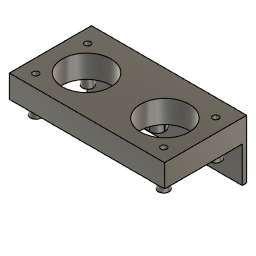
Chassis F360 (Autodesk Fusion 360 archive; units mm, degrees)
design "HC-SR04-UltrasonicSensor v7_Fitted Holes v8"
Autodesk Fusion 360 part; units mm, degrees
ref_plane "WorkPlane1" through (-22.725, -10, 13.61) normal (0, 0, 1) x (1, 0, 0)
sketch "Sketch1" plane through (0, 0, 13.61) normal (0, 0, 1) x (1, 0, 0)
  circle A0 centre (13.12, 0) radius 8
  circle A1 centre (-13.12, 0) radius 8
  circle A2 centre (-13.12, 0) radius 8.12
  circle A3 centre (13.12, 0) radius 8.12
  line L0 (26, -13) -> (-26, -13)
  line L1 (-26, -13) -> (-26, 13)
  line L2 (-26, 13) -> (26, 13)
  line L3 (26, 13) -> (26, -13)
  line L4 (26, -13) -> (-26, 13) construction
  line L5 (-26, -13) -> (26, 13) construction
  constraint concentric A1 A2
  constraint concentric A0 A3
  constraint horizontal L0
  constraint perpendicular L0 L1
  constraint parallel L0 L2
  constraint parallel L1 L3
  constraint coincident L4 origin
  constraint coincident L5 origin
extrude "Extrude1" add sketch "Sketch1" against normal blind 7.62 contours L0 L1 L2 L3
sketch "Sketch2" plane through (0, 0, 5.99) normal (0, 0, -1) x (-1, 0, 0)
  circle A0 centre (13.12, 0) radius 8.12
  circle A1 centre (-13.12, 0) radius 8.12
  line L0 (26, 13) -> (-26, 13)
  line L1 (-26, 13) -> (-26, -13)
  line L2 (-26, -13) -> (26, -13)
  line L3 (26, -13) -> (26, 13)
  arc A2 (5, 7.4356) -> (3.2, 9.2356) centre (3.2, 7.4356) ccw
  line L4 (5, 7.4356) -> (5, 7.3356)
  arc A3 (3.2, 5.5356) -> (5, 7.3356) centre (3.2, 7.3356) ccw
  line L5 (-3.2, 9.2356) -> (3.2, 9.2356)
  line L6 (3.2, 5.5356) -> (-3.2, 5.5356)
  arc A4 (-5, 7.3356) -> (-3.2, 5.5356) centre (-3.2, 7.3356) ccw
  line L7 (-5, 7.3356) -> (-5, 7.4356)
  arc A5 (-3.2, 9.2356) -> (-5, 7.4356) centre (-3.2, 7.4356) ccw
  line L8 (3.2, 9.2356) -> (-3.2, 9.2356)
  line L9 (3.2, 5.5356) -> (-3.2, 5.5356)
  arc A6 (5, 7.4356) -> (3.2, 9.2356) centre (3.2, 7.4356) ccw
  arc A7 (-3.2, 9.2356) -> (-5, 7.4356) centre (-3.2, 7.4356) ccw
  line L10 (5, 7.4356) -> (5, 7.3356)
  arc A8 (3.2, 5.5356) -> (5, 7.3356) centre (3.2, 7.3356) ccw
  arc A9 (-5, 7.3356) -> (-3.2, 5.5356) centre (-3.2, 7.3356) ccw
  line L11 (-5, 7.4356) -> (-5, 7.3356)
  line L12 (-5.1, 7.4356) -> (-5.1, 7.3356)
  arc A10 (-5.1, 7.3356) -> (-3.2, 5.4356) centre (-3.2, 7.3356) ccw
  line L13 (3.2, 5.4356) -> (-3.2, 5.4356)
  arc A11 (3.2, 5.4356) -> (5.1, 7.3356) centre (3.2, 7.3356) ccw
  line L14 (5.1, 7.4356) -> (5.1, 7.3356)
  arc A12 (5.1, 7.4356) -> (3.2, 9.3356) centre (3.2, 7.4356) ccw
  line L15 (3.2, 9.3356) -> (-3.2, 9.3356)
  arc A13 (-3.2, 9.3356) -> (-5.1, 7.4356) centre (-3.2, 7.4356) ccw
  line L16 (-5.7, 7.4356) -> (-5.7, 7.3356)
  arc A14 (-5.7, 7.3356) -> (-3.2, 4.8356) centre (-3.2, 7.3356) ccw
  line L17 (3.2, 4.8356) -> (-3.2, 4.8356)
  arc A15 (3.2, 4.8356) -> (5.7, 7.3356) centre (3.2, 7.3356) ccw
  line L18 (5.7, 7.4356) -> (5.7, 7.3356)
  arc A16 (5.7, 7.4356) -> (3.2, 9.9356) centre (3.2, 7.4356) ccw
  line L19 (3.2, 9.9356) -> (-3.2, 9.9356)
  arc A17 (-3.2, 9.9356) -> (-5.7, 7.4356) centre (-3.2, 7.4356) ccw
  circle A18 centre (21.425, -8.7) radius 1
  circle A19 centre (-21.425, -8.7) radius 1
  circle A20 centre (-21.425, 8.7) radius 1
  circle A21 centre (21.425, 8.7) radius 1
  circle A22 centre (-21.425, -8.7) radius 1.8
  circle A23 centre (-21.425, 8.7) radius 1.8
  circle A24 centre (21.425, 8.7) radius 1.8
  circle A25 centre (21.425, -8.7) radius 1.8
  point P0 (0, 7.3856)
  point P1 (0, 7.3856)
  dimension "d130" = 0.1
  dimension "d131" = 0.7
  dimension "d8" = 3.6
  dimension "d9" = 3.6
  dimension "d10" = 3.6
  dimension "d11" = 3.6
  dimension "d14" = 2
  dimension "d15" = 2
  dimension "d16" = 2
  dimension "d17" = 2
  constraint concentric A2 A6
  constraint concentric A5 A7
  constraint coincident A2.end L5.end
  constraint coincident L5.start A5.start
  constraint coincident A3.start L6.start
  constraint coincident L6.end A4.end
  constraint coincident A2.start L4.start
  constraint coincident L4.end A3.end
  constraint tangent L6 A8
  constraint tangent L4 A8
  constraint tangent L6 A9
  constraint tangent L7 A9
  constraint coincident L7.end A5.end
  constraint tangent A4 L11
  constraint coincident P1 P0
  constraint concentric A20 A23
  constraint concentric A21 A24
  constraint concentric A18 A25
  measures "d130" distance of L11
  measures "d8" diameter of A22
  measures "d9" diameter of A23
  measures "d10" diameter of A24
  measures "d11" diameter of A25
  measures "d14" diameter of A20
  measures "d15" diameter of A21
  measures "d16" diameter of A18
  measures "d17" diameter of A19
extrude "Extrude2" add sketch "Sketch2" along normal blind 3.69 contours L16 A14 L17 A15 L18 A16 L19 A17
sketch "Sketch3" plane through (0, 0, 5.99) normal (0, 0, -1) x (-1, 0, 0)
extrude "Extrude4" cut sketch "Sketch2" against normal through all contours A18 | A19 | A20 | A21
extrude "Extrude6" add sketch "Sketch2" along normal blind 4.38 contours A22 | A23 | A24 | A25
sketch "Sketch4" plane through (0, 13, 0) normal (0, 1, 0) x (-1, 0, 0)
  line L0 (26, 13.61) -> (-26, 13.61)
  line L1 (-26, 13.61) -> (-26, 5.99)
  line L2 (-26, 5.99) -> (26, 5.99)
  line L3 (26, 5.99) -> (26, 13.61)
  line L4 (26, -6.01) -> (-26, -6.01)
  line L5 (-26, -6.01) -> (-26, 25.61)
  line L6 (-26, 25.61) -> (26, 25.61)
  line L7 (26, 25.61) -> (26, -6.01)
  line L8 (5, 5.99) -> (21.24, 5.99)
  dimension "d18" = 12
  dimension "d19" = 12
  constraint horizontal L4
  constraint vertical L5
  constraint horizontal L6
  constraint vertical L7
  measures "d18" distance of L4 L8
  measures "d19" distance of L0 L6
extrude "Extrude7" add sketch "Sketch4" along normal blind 1.5
extrude "Extrude8" cut 1 faces at (8.6667, 13.5, 25.61) along direction (0, 0, -1) up to surface (12 mm away)

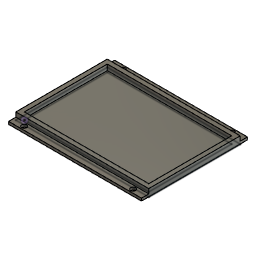
design "BreadBoard Mount"
Autodesk Fusion 360 part; units mm, degrees
sketch "Sketch1" plane through (0, 0, 0) normal (0, 1, 0) x (1, 0, 0)
  line L0 (0, 0) -> (87, 0)
  line L1 (87, 0) -> (87, 58)
  line L2 (87, 58) -> (0, 58)
  line L3 (0, 58) -> (0, 0)
  line L4 (-3, 61) -> (90, 61)
  line L5 (90, 61) -> (90, -3)
  line L6 (90, -3) -> (-3, -3)
  line L7 (-3, -3) -> (-3, 61)
  dimension "d1" = 87
  dimension "d2" = 58
  dimension "d3" = 3
  dimension "d4" = 3
  dimension "d5" = 3
  dimension "d6" = 3
  constraint horizontal L0
  constraint vertical L1
  constraint horizontal L2
  constraint vertical L3
  constraint coincident L0.start L3.end
  constraint horizontal L4
  constraint vertical L5
  constraint horizontal L6
  constraint vertical L7
  measures "d1" distance of L0.start L0.end
  measures "d2" distance of L0.start L2.end
  measures "d3" distance of L1 L5
  measures "d4" distance of L0 L6
  measures "d5" distance of L3 L7
  measures "d6" distance of L2 L4
extrude "Extrude1" add sketch "Sketch1" along normal blind 5
extrude "Extrude2" add sketch "Sketch1" along normal blind 1 contours L0 L1 L2 L3
sketch "Sketch2" plane through (0, 0, 0) normal (0, 1, 0) x (1, 0, 0)
  line L0 (90, -3) -> (-3, -3)
  line L1 (-3, -3) -> (-3, 61)
  line L2 (-3, 61) -> (90, 61)
  line L3 (90, 61) -> (90, -3)
  circle A0 centre (81.6, 63.54) radius 1.75
  circle A1 centre (5.4, 63.54) radius 1.75
  line L4 (-3, -3) -> (-3, 61)
  line L5 (-3, 61) -> (90, 61)
  circle A2 centre (81.6, -5.54) radius 1.75
  circle A3 centre (5.4, -5.54) radius 1.75
  line L6 (90, -3) -> (-3, -3)
  line L7 (-3, 66.08) -> (90, 66.08)
  line L8 (90, 66.08) -> (90, -8.08)
  line L9 (90, -8.08) -> (-3, -8.08)
  line L10 (-3, -8.08) -> (-3, 66.08)
  dimension "d11" = 3.5
  dimension "d12" = 3.5
  dimension "d13" = 76.2
  dimension "d14" = 8.4
  dimension "d15" = 2.54
  dimension "d16" = 3.5
  dimension "d17" = 3.5
  dimension "d18" = 2.54
  dimension "d19" = 2.54
  dimension "d21" = 2.54
  dimension "d22" = 2.54
  constraint horizontal L7
  constraint vertical L8
  constraint horizontal L9
  constraint vertical L10
  measures "d11" diameter of A0
  measures "d12" diameter of A1
  measures "d13" distance of A0.centre A1.centre
  measures "d14" distance of A1.centre L4
  measures "d15" distance of A0.centre L5
  measures "d16" diameter of A2
  measures "d17" diameter of A3
  measures "d18" distance of A3.centre L6
  measures "d19" distance of A2.centre L6
  measures "d21" distance of A3.centre L9
  measures "d22" distance of A0.centre L7
extrude "Extrude3" add sketch "Sketch2" along normal blind 1.778 contours L0 L6 L8 L9 L10 | L2 L5 L7 L8 L10
equation "d4 = d3"
equation "d5 = d4"

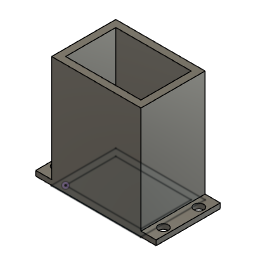
design "NewBatteryMount"
Autodesk Fusion 360 part; units mm, degrees
sketch "Sketch1" plane through (0, 0, 0) normal (0, 1, 0) x (1, 0, 0)
  line L0 (0, 0) -> (27, 0)
  line L1 (27, 0) -> (27, 18)
  line L2 (27, 18) -> (0, 18)
  line L3 (0, 18) -> (0, 0)
  line L4 (-2.5, 20.5) -> (29.5, 20.5)
  line L5 (29.5, 20.5) -> (29.5, -2.5)
  line L6 (29.5, -2.5) -> (-2.5, -2.5)
  line L7 (-2.5, -2.5) -> (-2.5, 20.5)
  dimension "d1" = 27
  dimension "d2" = 18
  dimension "d3" = 2.5
  dimension "d4" = 2.5
  dimension "d5" = 2.5
  dimension "d6" = 2.5
  constraint horizontal L0
  constraint vertical L1
  constraint horizontal L2
  constraint vertical L3
  constraint coincident L0.start L3.end
  constraint horizontal L4
  constraint vertical L5
  constraint horizontal L6
  constraint vertical L7
  measures "d1" distance of L0.start L0.end
  measures "d2" distance of L0.start L2.end
  measures "d3" distance of L0 L6
  measures "d4" distance of L1 L5
  measures "d5" distance of L3 L7
  measures "d6" distance of L2 L4
extrude "Extrude1" add sketch "Sketch1" along normal blind 40
extrude "Extrude2" add sketch "Sketch1" along normal blind 2.5 contours L0 L1 L2 L3
sketch "Sketch2" plane through (0, 0, 0) normal (0, 1, 0) x (1, 0, 0)
  circle A0 centre (-5.6754, 2.65) radius 1.75
  circle A1 centre (32.4246, 2.65) radius 1.75
  line L0 (29.5, -2.5) -> (-2.5, -2.5)
  circle A2 centre (-5.6754, 15.35) radius 1.75
  circle A3 centre (32.4246, 15.35) radius 1.75
  line L1 (29.5, -2.5) -> (-2.5, -2.5)
  line L2 (-2.5, -2.5) -> (-2.5, 20.5)
  line L3 (-2.5, 20.5) -> (29.5, 20.5)
  line L4 (29.5, 20.5) -> (29.5, -2.5)
  line L5 (-8.2154, -2.5) -> (34.9646, -2.5)
  line L6 (34.9646, -2.5) -> (34.9646, 20.5)
  line L7 (34.9646, 20.5) -> (-8.2154, 20.5)
  line L8 (-8.2154, 20.5) -> (-8.2154, -2.5)
  dimension "d11" = 3.5
  dimension "d12" = 3.5
  dimension "d13" = 38.1
  dimension "d15" = 5.15
  dimension "d16" = 3.5
  dimension "d17" = 12.7
  dimension "d18" = 3.5
  dimension "d19" = 2.54
  dimension "d20" = 2.54
  constraint horizontal L5
  constraint vertical L6
  constraint horizontal L7
  constraint vertical L8
  measures "d11" diameter of A0
  measures "d12" diameter of A1
  measures "d13" distance of A0.centre A1.centre
  measures "d15" distance of A0.centre L0
  measures "d16" diameter of A2
  measures "d17" distance of A0.centre A2.centre
  measures "d18" diameter of A3
  measures "d19" distance of A0.centre L8
  measures "d20" distance of A1.centre L6
extrude "Extrude3" add sketch "Sketch2" along normal blind 1.778 contours L4 L5 L6 L7 | L2 L5 L7 L8
equation "d4 = d3"
equation "d5 = d3"
equation "d6 = d3"
